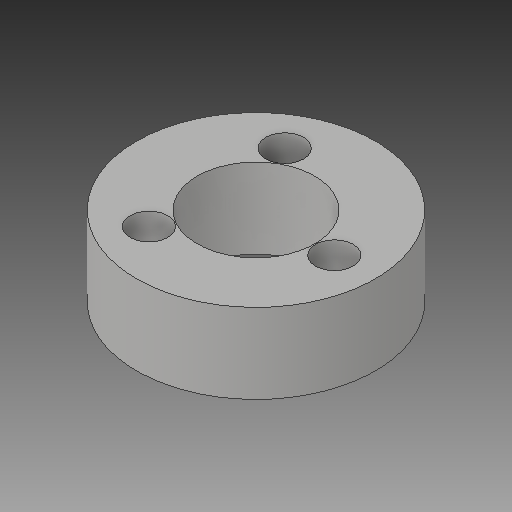
# Autodesk Inventor part: chuck holder
Saved by Autodesk Inventor 2018 (Build 220112000, 112)
## iProperties
Created: 2017-06-20
Part Number: chuck holder
Material: Generic
Document SubType Name: Modeling
Designer: M228854
Density: 1 g/cm^3
Appearance: Default
Mass: 310.318 g
Surface Area: 452.403 cm^2
Volume: 310.318 cm^3
Author: M228854
Autodesk Inventor part; units mm, degrees
ref_plane "YZ Plane" through (0, 0, 0) normal (1, 0, 0) x (0, 1, 0)
ref_plane "XZ Plane" through (0, 0, 0) normal (0, 1, 0) x (-1, 0, 0)
ref_plane "XY Plane" through (0, 0, 0) normal (0, 0, 1) x (1, 0, 0)
sketch "Sketch1" plane through (0, 0, 0) normal (0, 1, 0) x (-1, 0, 0)
  circle A0 centre (0, 0) radius 60.05
  circle A1 centre (0, 0) radius 29.55
  constraints: 2 centre point, 2 coincident
extrude "Extrusion1" add sketch "Sketch1" along normal blind 40.12
sketch "Sketch2" plane through (0, 40.12, 0) normal (0, 1, 0) x (1, 0, 0)
  circle A0 centre (0, 0) radius 29.55 projected
  circle A1 centre (39.43, 0) radius 9.5
  circle A2 centre (-19.715, 34.1474) radius 9.5
  circle A3 centre (-19.715, -34.1474) radius 9.5
  dimension "d13" = 360
  constraints: 3 centre point, 7 other
extrude "Extrusion2" cut sketch "Sketch2" against normal blind 40.12 contours A1 | A2 | A3
body "Solid1"
